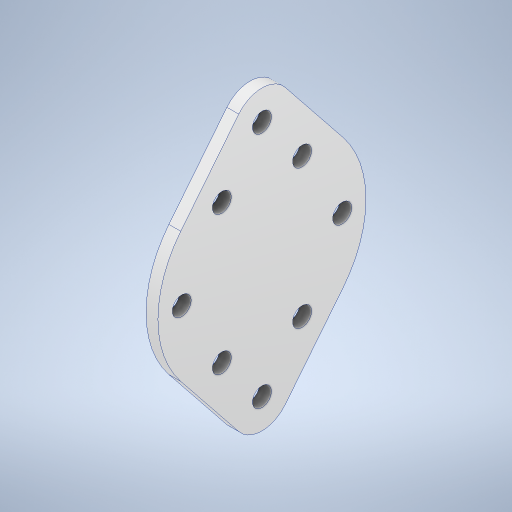
# Autodesk Inventor part: endeff_plate2
Saved by Autodesk Inventor 2024 (Build 280153000, 153)
## iProperties
Created: 2024-12-13
Part Number: endeff_plate2
Material: アルミニウム 6061
Document SubType Name: Modeling
Designer: hirek
Density: 2.7 g/cm^3
Appearance: アルミニウム - フラット
Author: hirek
Autodesk Inventor part; units mm, degrees
ref_plane "YZ Plane" through (0, 0, 0) normal (1, 0, 0) x (0, 1, 0)
ref_plane "XZ Plane" through (0, 0, 0) normal (0, 1, 0) x (-1, 0, 0)
ref_plane "XY Plane" through (0, 0, 0) normal (0, 0, 1) x (1, 0, 0)
sketch "スケッチ1" plane through (0, 0, 0) normal (1, 0, 0) x (0, 1, 0)
  circle A0 centre (0, 0) radius 17.5
  dimension "d0" = 35
  constraints: 1 centre point, 1 coincident
  measures "d0" diameter of A0
extrude "押し出し1" add sketch "スケッチ1" along normal blind 3
sketch "スケッチ2" plane through (3, 0, 0) normal (1, 0, 0) x (0, 0, -1)
  circle A0 centre (0, 0) radius 13.5
  point P0 (13.5, 0)
  point P1 (6.75, 11.6913)
  point P2 (-6.75, 11.6913)
  point P3 (-13.5, 0)
  point P4 (-6.75, -11.6913)
  point P5 (6.75, -11.6913)
  dimension "d3" = 27
  dimension "d6" = 360
  constraints: 1 coincident, 1 horizontal alignment, 9 other
hole "穴1" at (3, 0, -13.5) at (3, 11.6913, -6.75) at (3, 11.6913, 6.75) at (3, 0, 13.5) at (3, -11.6913, 6.75) at (3, -11.6913, -6.75) direction (-1, 0, 0) diameter 3.2 end through all
sketch "スケッチ4" plane through (3, 0, 0) normal (1, 0, 0) x (0, 0, -1)
  circle A0 centre (0, 0) radius 20
  circle A1 centre (0, -20) radius 5
  circle A2 centre (0, 20) radius 5
  circle A3 centre (13.5, 0) radius 1.6 projected
  circle A4 centre (-13.5, 0) radius 1.6 projected
  line L0 (-24.9861, -3.2077) -> (0.509, 28.6357)
  line L1 (1.3172, 26.3548) -> (24.4586, -2.5487)
  line L2 (-28.3137, 7.3638) -> (1.2125, -29.5144)
  line L3 (-0.4955, -28.6189) -> (23.5579, 1.4238)
  circle A5 centre (0, 0) radius 17.5 projected
  point P0 (-3.9031, 23.125)
  point P1 (-13.6609, 10.9375)
  point P2 (-13.6609, -10.9375)
  point P3 (-3.9031, -23.125)
  point P4 (3.9031, -23.125)
  point P5 (13.6609, -10.9375)
  point P6 (13.6609, 10.9375)
  point P7 (3.9031, 23.125)
  dimension "d22" = 40
  dimension "d23" = 10
  dimension "d24" = 10
  dimension "d25" = 13.5
  dimension "d26" = 13.5
  constraints: 8 end point, 8 tangent, 3 centre point, 2 point on circle, 1 coincident
  measures "d22" diameter of A0
  measures "d23" diameter of A1
  measures "d24" diameter of A2
  measures "d25" horizontal distance of A2.centre A3.centre
  measures "d26" horizontal distance of A1.centre A4.centre
extrude "押し出し2" add sketch "スケッチ4" against normal blind 2 contours L1 A5 A2 A0 | A0 A2 L1 | A5 A1 A2 | L3 A1 A0 | A0 A1 A5 L3 | A2 A5 A0 | A0 A2 | A2 A5 | A1 A0 | A0 A1 A5 | A5 A1 | A2 A5 L0 A0 | A0 L0 A2 | A1 L2 A0 | A0 L2 A5 A1
sketch "スケッチ5" plane through (0, 0, 0) normal (-1, 0, 0) x (0, 0, 1)
  circle A0 centre (6.75, -11.6913) radius 1.6 projected
  circle A1 centre (-6.75, -11.6913) radius 1.6 projected
  circle A2 centre (-6.75, 11.6913) radius 1.6 projected
  circle A3 centre (6.75, 11.6913) radius 1.6 projected
  arc A4 (3.9031, 23.125) -> (-3.9031, 23.125) centre (0, 20) ccw projected
  arc A5 (-3.9031, -23.125) -> (3.9031, -23.125) centre (0, -20) ccw projected
  point P0 (0, 0)
  constraints: 6 coincident
hole "穴2" at (0, -11.6913, 6.75) at (0, -11.6913, -6.75) at (0, 11.6913, -6.75) at (0, 11.6913, 6.75) at (0, 20, 0) at (0, -20, 0) direction (1, 0, 0) diameter 3.2 depth 5
sketch "スケッチ6" plane through (0, 0, 0) normal (-1, 0, 0) x (0, 0, 1)
  circle A0 centre (0, 0) radius 17.5
  constraints: 1 centre point, 1 coincident
extrude "押し出し3" cut sketch "スケッチ6" against normal blind 1
